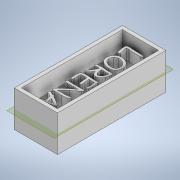
# Autodesk Inventor part: Pieza2
Saved by Autodesk Inventor 2021 (Build 250183000, 183)
## iProperties
Created: 2022-09-17
Part Number: Pieza2
Material: Genérico
Document SubType Name: Modeling
Designer: sergi
Density: 1 g/cm^3
Appearance: Valor por defecto
Author: sergi
Autodesk Inventor part; units mm, degrees
ref_plane "YZ Plane" through (0, 0, 0) normal (1, 0, 0) x (0, 1, 0)
ref_plane "XZ Plane" through (0, 0, 0) normal (0, 1, 0) x (-1, 0, 0)
ref_plane "XY Plane" through (0, 0, 0) normal (0, 0, 1) x (1, 0, 0)
sketch "Boceto1" plane through (0, 0, 0) normal (0, 1, 0) x (-1, 0, 0)
  line L0 (-6, -15) -> (6, -15)
  line L1 (6, -15) -> (6, 15)
  line L2 (6, 15) -> (-6, 15)
  line L3 (-6, 15) -> (-6, -15)
  line L4 (-6, -15) -> (6, 15) construction
  line L5 (6, -15) -> (-6, 15) construction
  line L6 (6, 15) -> (6, -15) construction
  line L7 (6, -15) -> (-6, -15) construction
  line L8 (-6, -15) -> (-6, 15) construction
  line L9 (-6, 15) -> (6, 15) construction
  point P0 (0, 0)
  dimension "d0" = 12
  dimension "d1" = 30
  dimension "d9" = 30
  dimension "d10" = 12
  constraints: 12 end point, 2 midpoint, 2 parallel, 1 horizontal, 1 perpendicular, 2 other
  measures "d0" distance of L2.end L1.end
  measures "d1" distance of L1.end L0.end
  measures "d9" distance of L7.end L9.start
  measures "d10" distance of L6.end L7.end
extrude "Extrusión1" add sketch "Boceto1" along normal blind 10
shell "Vaciado1" thickness 1 removed faces 1 at (2, 10, -5) ; own thickness 5 on faces at (2, 0, -5) ; own thickness 1 on faces at (2, 3.3333, -15)
sketch "Boceto2" plane through (-5, 5, 14) normal (0, 1, 0) x (1, 0, 0)
  line L0 (10.9835, 29) -> (10.9835, -1) construction
  line L1 (10.9835, -1) -> (-1.0165, -1) construction
  line L2 (-1.0165, -1) -> (-1.0165, 29) construction
  line L3 (-1.0165, 29) -> (10.9835, 29) construction
  line L4 (0, -2.0428) -> (0, 28)
  line L5 (-1, -1) -> (11, -1) projected
  spline S0 degree 2 poles (2.781, 23.9073) (2.6172, 24.2565) (2.4879, 25.0065) knots 0 0 0 1 1 1
  spline S1 degree 2 poles (2.4879, 25.0065) (2.3672, 25.6961) (2.3672, 26.1315) knots 0 0 0 1 1 1
  spline S2 degree 2 poles (2.3672, 26.1315) (2.3672, 26.4418) (2.462, 26.5797) knots 0 0 0 1 1 1
  spline S3 degree 2 poles (2.462, 26.5797) (2.5913, 26.7651) (2.9404, 26.7651) knots 0 0 0 1 1 1
  line L6 (2.9404, 26.7651) -> (3.962, 26.7047)
  spline S4 degree 2 poles (3.962, 26.7047) (5.3801, 26.6228) (7.1042, 26.6228) knots 0 0 0 1 1 1
  spline S5 degree 2 poles (7.1042, 26.6228) (7.2379, 26.6228) (7.4232, 26.4461) (7.4232, 26.3168) knots 0 0 0 1 2 2 2
  spline S6 degree 2 poles (7.4232, 26.3168) (7.4232, 26.1832) (7.2379, 26.0065) (7.1042, 26.0065) knots 0 0 0 1 2 2 2
  spline S7 degree 2 poles (7.1042, 26.0065) (5.3585, 26.0065) (3.9275, 26.0884) knots 0 0 0 1 1 1
  line L7 (3.9275, 26.0884) -> (3.4534, 26.1315)
  spline S8 degree 2 poles (3.4534, 26.1315) (3.1991, 26.153) (3.0008, 26.1487) knots 0 0 0 1 1 1
  spline S9 degree 2 poles (3.0008, 26.1487) (2.9922, 25.3427) (3.3758, 24.1099) knots 0 0 0 1 1 1
  spline S10 degree 2 poles (3.3758, 24.1099) (3.393, 24.0539) (3.393, 24.0108) knots 0 0 0 1 1 1
  spline S11 degree 2 poles (3.393, 24.0108) (3.393, 23.8772) (3.2896, 23.7866) knots 0 0 0 1 1 1
  spline S12 degree 2 poles (3.2896, 23.7866) (3.1948, 23.7091) (3.0698, 23.7091) knots 0 0 0 1 1 1
  spline S13 degree 2 poles (3.0698, 23.7091) (2.8715, 23.7091) (2.781, 23.9073) knots 0 0 0 1 1 1
  spline S14 degree 2 poles (2.4663, 21.1099) (2.4663, 21.9806) (2.9879, 22.5884) knots 0 0 0 1 1 1
  spline S15 degree 2 poles (2.9879, 22.5884) (3.5439, 23.2306) (4.4232, 23.2306) knots 0 0 0 1 1 1
  spline S16 degree 2 poles (4.4232, 23.2306) (5.4965, 23.2306) (6.3715, 22.597) knots 0 0 0 1 1 1
  spline S17 degree 2 poles (6.3715, 22.597) (7.3413, 21.8901) (7.3413, 20.8297) knots 0 0 0 1 1 1
  spline S18 degree 2 poles (7.3413, 20.8297) (7.3413, 19.8168) (6.8844, 19.3211) knots 0 0 0 1 1 1
  spline S19 degree 2 poles (6.8844, 19.3211) (6.406, 18.8039) (5.3801, 18.8039) knots 0 0 0 1 1 1
  spline S20 degree 2 poles (5.3801, 18.8039) (4.3111, 18.8039) (3.4491, 19.3858) knots 0 0 0 1 1 1
  spline S21 degree 2 poles (3.4491, 19.3858) (2.4663, 20.0539) (2.4663, 21.1099) knots 0 0 0 1 1 1
  spline S22 degree 2 poles (6.7077, 20.8297) (6.7077, 21.5884) (5.9534, 22.1142) knots 0 0 0 1 1 1
  spline S23 degree 2 poles (5.9534, 22.1142) (5.2594, 22.6013) (4.4232, 22.6013) knots 0 0 0 1 1 1
  spline S24 degree 2 poles (4.4232, 22.6013) (3.8284, 22.6013) (3.4534, 22.1573) knots 0 0 0 1 1 1
  spline S25 degree 2 poles (3.4534, 22.1573) (3.0999, 21.7349) (3.0999, 21.1099) knots 0 0 0 1 1 1
  spline S26 degree 2 poles (3.0999, 21.1099) (3.0999, 20.3599) (3.8585, 19.8685) knots 0 0 0 1 1 1
  spline S27 degree 2 poles (3.8585, 19.8685) (4.5353, 19.4332) (5.3801, 19.4332) knots 0 0 0 1 1 1
  spline S28 degree 2 poles (5.3801, 19.4332) (6.1215, 19.4332) (6.4189, 19.7651) knots 0 0 0 1 1 1
  spline S29 degree 2 poles (6.4189, 19.7651) (6.7077, 20.0797) (6.7077, 20.8297) knots 0 0 0 1 1 1
  spline S30 degree 2 poles (2.6215, 15.0496) (2.6215, 15.1659) (2.7206, 15.2694) knots 0 0 0 1 1 1
  spline S31 degree 2 poles (2.7206, 15.2694) (3.7292, 16.2909) (4.0784, 17.5453) knots 0 0 0 1 1 1
  line L8 (4.0784, 17.5453) -> (3.4749, 17.5194)
  line L9 (3.4749, 17.5194) -> (2.8672, 17.5022)
  spline S32 degree 2 poles (2.8672, 17.5022) (2.7292, 17.5022) (2.5482, 17.6789) (2.5482, 17.8125) knots 0 0 0 1 2 2 2
  spline S33 degree 2 poles (2.5482, 17.8125) (2.5482, 17.9461) (2.7292, 18.1228) (2.8672, 18.1228) knots 0 0 0 1 2 2 2
  spline S34 degree 2 poles (2.8672, 18.1228) (3.1129, 18.1228) (4.0784, 18.1703) (4.3241, 18.1703) knots 0 0 0 1 2 2 2
  spline S35 degree 2 poles (4.3241, 18.1703) (4.6085, 18.1703) (5.7335, 18.0453) (6.0137, 18.0453) knots 0 0 0 1 2 2 2
  spline S36 degree 2 poles (6.0137, 18.0453) (6.1732, 18.0453) (6.7896, 18.1056) (6.9491, 18.1056) knots 0 0 0 1 2 2 2
  spline S37 degree 2 poles (6.9491, 18.1056) (7.1258, 18.1056) (7.2594, 18.0065) knots 0 0 0 1 1 1
  spline S38 degree 2 poles (7.2594, 18.0065) (7.4232, 17.8901) (7.406, 17.6832) knots 0 0 0 1 1 1
  line L10 (7.406, 17.6832) -> (7.3456, 16.9375)
  spline S39 degree 2 poles (7.3456, 16.9375) (7.2939, 16.5151) (7.1387, 16.222) knots 0 0 0 1 1 1
  spline S40 degree 2 poles (7.1387, 16.222) (6.4749, 14.972) (5.518, 14.972) knots 0 0 0 1 1 1
  spline S41 degree 2 poles (5.518, 14.972) (5.0482, 14.972) (4.6861, 15.3987) knots 0 0 0 1 1 1
  spline S42 degree 2 poles (4.6861, 15.3987) (4.393, 15.7392) (4.2422, 16.2522) knots 0 0 0 1 1 1
  spline S43 degree 2 poles (4.2422, 16.2522) (3.7249, 15.2909) (3.1516, 14.8168) knots 0 0 0 1 1 1
  spline S44 degree 2 poles (3.1516, 14.8168) (3.0525, 14.7349) (2.9448, 14.7349) knots 0 0 0 1 1 1
  spline S45 degree 2 poles (2.9448, 14.7349) (2.8111, 14.7349) (2.6215, 14.9246) (2.6215, 15.0496) knots 0 0 0 1 2 2 2
  line L11 (6.7077, 17.0194) -> (6.7465, 17.4763)
  line L12 (6.7465, 17.4763) -> (6.3715, 17.4461)
  spline S46 degree 2 poles (6.3715, 17.4461) (6.143, 17.4246) (5.9965, 17.4246) knots 0 0 0 1 1 1
  spline S47 degree 2 poles (5.9965, 17.4246) (5.7508, 17.4246) (5.3801, 17.4634) knots 0 0 0 1 1 1
  line L13 (5.3801, 17.4634) -> (4.7637, 17.528)
  spline S48 degree 2 poles (4.7637, 17.528) (4.7637, 17.4849) (4.7594, 17.3039) (4.7594, 17.2565) knots 0 0 0 1 2 2 2
  spline S49 degree 2 poles (4.7594, 17.2565) (4.7594, 16.4677) (4.9706, 16.0754) knots 0 0 0 1 1 1
  spline S50 degree 2 poles (4.9706, 16.0754) (5.0654, 15.903) (5.2206, 15.7565) knots 0 0 0 1 1 1
  spline S51 degree 2 poles (5.2206, 15.7565) (5.393, 15.5927) (5.5137, 15.5927) knots 0 0 0 1 1 1
  spline S52 degree 2 poles (5.5137, 15.5927) (5.9448, 15.5927) (6.3154, 16.0797) knots 0 0 0 1 1 1
  spline S53 degree 2 poles (6.3154, 16.0797) (6.656, 16.528) (6.7077, 17.0194) knots 0 0 0 1 1 1
  spline S54 degree 2 poles (6.8154, 11.1056) (6.8154, 11.1487) (6.8327, 11.2047) knots 0 0 0 1 1 1
  spline S55 degree 2 poles (6.8327, 11.2047) (6.9792, 11.7263) (6.9792, 12.2134) knots 0 0 0 1 1 1
  spline S56 degree 2 poles (6.9792, 12.2134) (6.9792, 12.4634) (6.8887, 13.0668) (6.7939, 13.4116) knots 0 0 0 1 2 2 2
  spline S57 degree 2 poles (6.7939, 13.4116) (6.5913, 13.3815) (6.4706, 13.3815) knots 0 0 0 1 1 1
  spline S58 degree 2 poles (6.4706, 13.3815) (6.0439, 13.3815) (5.2896, 13.4375) knots 0 0 0 1 1 1
  line L14 (5.2896, 13.4375) -> (5.4189, 12.0797)
  spline S59 degree 2 poles (5.4189, 12.0797) (5.4792, 11.4849) (5.4792, 11.3513) knots 0 0 0 1 1 1
  spline S60 degree 2 poles (5.4792, 11.3513) (5.4792, 11.2134) (5.3068, 11.028) (5.1603, 11.028) knots 0 0 0 1 2 2 2
  spline S61 degree 2 poles (5.1603, 11.028) (4.8801, 11.028) (4.8456, 11.3125) knots 0 0 0 1 1 1
  line L15 (4.8456, 11.3125) -> (4.781, 12.0496)
  line L16 (4.781, 12.0496) -> (4.6516, 13.4806)
  spline S62 degree 2 poles (4.6516, 13.4806) (4.4318, 13.4935) (4.0396, 13.5065) (3.8715, 13.5065) knots 0 0 0 1 2 2 2
  spline S63 degree 2 poles (3.8715, 13.5065) (3.1861, 13.5065) (3.0654, 13.4073) knots 0 0 0 1 1 1
  spline S64 degree 2 poles (3.0654, 13.4073) (2.9792, 13.3341) (2.9792, 12.9203) knots 0 0 0 1 1 1
  spline S65 degree 2 poles (2.9792, 12.9203) (2.9792, 12.7306) (3.0008, 11.9591) (3.0008, 11.7651) knots 0 0 0 1 2 2 2
  spline S66 degree 2 poles (3.0008, 11.7651) (3.0008, 11.7047) (3.0396, 11.4634) (3.0396, 11.403) knots 0 0 0 1 2 2 2
  spline S67 degree 2 poles (3.0396, 11.403) (3.0396, 11.0754) (2.7206, 11.0754) knots 0 0 0 1 1 1
  spline S68 degree 2 poles (2.7206, 11.0754) (2.462, 11.0754) (2.4103, 11.3384) knots 0 0 0 1 1 1
  spline S69 degree 2 poles (2.4103, 11.3384) (2.3499, 11.6272) (2.3499, 12.597) knots 0 0 0 1 1 1
  spline S70 degree 2 poles (2.3499, 12.597) (2.3499, 13.5539) (2.6042, 13.8254) knots 0 0 0 1 1 1
  spline S71 degree 2 poles (2.6042, 13.8254) (2.8801, 14.1228) (3.8715, 14.1228) knots 0 0 0 1 1 1
  spline S72 degree 2 poles (3.8715, 14.1228) (4.0698, 14.1228) (4.5396, 14.1056) (4.8111, 14.0884) knots 0 0 0 1 2 2 2
  spline S73 degree 2 poles (4.8111, 14.0884) (4.8801, 14.1228) (4.962, 14.1228) knots 0 0 0 1 1 1
  spline S74 degree 2 poles (4.962, 14.1228) (5.0654, 14.1228) (5.1516, 14.0625) knots 0 0 0 1 1 1
  spline S75 degree 2 poles (5.1516, 14.0625) (6.0439, 14.0022) (6.4706, 14.0022) knots 0 0 0 1 1 1
  spline S76 degree 2 poles (6.4706, 14.0022) (6.587, 14.0022) (7.0266, 14.0625) (7.143, 14.0625) knots 0 0 0 1 2 2 2
  spline S77 degree 2 poles (7.143, 14.0625) (7.5094, 14.0625) (7.5094, 13.7522) knots 0 0 0 1 1 1
  spline S78 degree 2 poles (7.5094, 13.7522) (7.5094, 13.6228) (7.4189, 13.5323) knots 0 0 0 1 1 1
  spline S79 degree 2 poles (7.4189, 13.5323) (7.518, 13.1616) (7.6172, 12.5022) (7.6172, 12.2091) knots 0 0 0 1 2 2 2
  spline S80 degree 2 poles (7.6172, 12.2091) (7.6172, 11.4591) (7.4361, 11.0108) knots 0 0 0 1 1 1
  spline S81 degree 2 poles (7.4361, 11.0108) (7.3542, 10.8039) (7.1387, 10.8039) knots 0 0 0 1 1 1
  spline S82 degree 2 poles (7.1387, 10.8039) (7.018, 10.8039) (6.9189, 10.8858) knots 0 0 0 1 1 1
  spline S83 degree 2 poles (6.9189, 10.8858) (6.8154, 10.972) (6.8154, 11.1056) knots 0 0 0 1 1 1
  spline S84 degree 2 poles (3.3413, 5.8341) (3.1948, 5.8341) (2.8456, 5.8858) knots 0 0 0 1 1 1
  spline S85 degree 2 poles (2.8456, 5.8858) (2.5353, 5.9332) (2.5353, 6.2134) knots 0 0 0 1 1 1
  spline S86 degree 2 poles (2.5353, 6.2134) (2.5353, 6.3858) (2.7594, 6.6228) knots 0 0 0 1 1 1
  spline S87 degree 2 poles (2.7594, 6.6228) (3.9491, 7.8772) (6.1948, 9.5065) knots 0 0 0 1 1 1
  line L17 (6.1948, 9.5065) -> (5.4922, 9.5237)
  line L18 (5.4922, 9.5237) -> (4.7853, 9.5323)
  spline S88 degree 2 poles (4.7853, 9.5323) (4.531, 9.5323) (3.5008, 9.5108) (3.2422, 9.5108) knots 0 0 0 1 2 2 2
  spline S89 degree 2 poles (3.2422, 9.5108) (2.4103, 9.5108) (2.4103, 9.8341) knots 0 0 0 1 1 1
  spline S90 degree 2 poles (2.4103, 9.8341) (2.4103, 10.0022) (2.518, 10.1013) knots 0 0 0 1 1 1
  spline S91 degree 2 poles (2.518, 10.1013) (2.6129, 10.1918) (2.7465, 10.1918) knots 0 0 0 1 1 1
  spline S92 degree 2 poles (2.7465, 10.1918) (2.8758, 10.1918) (3.4016, 10.153) (3.5353, 10.153) knots 0 0 0 1 2 2 2
  spline S93 degree 2 poles (3.5353, 10.153) (3.7249, 10.153) (4.4879, 10.1272) (4.6818, 10.1272) knots 0 0 0 1 2 2 2
  spline S94 degree 2 poles (4.6818, 10.1272) (4.8844, 10.1272) (5.712, 10.1444) (5.9146, 10.1444) knots 0 0 0 1 2 2 2
  spline S95 degree 2 poles (5.9146, 10.1444) (6.1085, 10.1444) (6.8801, 10.222) (7.0741, 10.222) knots 0 0 0 1 2 2 2
  spline S96 degree 2 poles (7.0741, 10.222) (7.2163, 10.222) (7.4534, 9.9763) (7.4534, 9.8211) knots 0 0 0 1 2 2 2
  spline S97 degree 2 poles (7.4534, 9.8211) (7.4534, 9.6573) (7.0956, 9.4159) knots 0 0 0 1 1 1
  spline S98 degree 2 poles (7.0956, 9.4159) (5.9404, 8.6444) (5.1775, 8.0323) knots 0 0 0 1 1 1
  spline S99 degree 2 poles (5.1775, 8.0323) (4.2723, 7.2996) (3.4448, 6.4246) knots 0 0 0 1 1 1
  spline S100 degree 2 poles (3.4448, 6.4246) (3.5784, 6.4159) (3.837, 6.4246) knots 0 0 0 1 1 1
  line L19 (3.837, 6.4246) -> (4.2249, 6.4332)
  spline S101 degree 2 poles (4.2249, 6.4332) (5.5827, 6.4332) (6.3887, 6.5366) knots 0 0 0 1 1 1
  spline S102 degree 2 poles (6.3887, 6.5366) (6.4663, 6.5496) (6.712, 6.6228) knots 0 0 0 1 1 1
  spline S103 degree 2 poles (6.712, 6.6228) (6.9232, 6.6832) (7.0396, 6.6832) knots 0 0 0 1 1 1
  spline S104 degree 2 poles (7.0396, 6.6832) (7.3973, 6.6832) (7.3973, 6.3556) knots 0 0 0 1 1 1
  spline S105 degree 2 poles (7.3973, 6.3556) (7.3973, 5.8168) (5.393, 5.8168) knots 0 0 0 1 1 1
  spline S106 degree 2 poles (5.393, 5.8168) (5.0482, 5.8168) (3.6861, 5.8341) (3.3413, 5.8341) knots 0 0 0 1 2 2 2
  spline S107 degree 2 poles (2.5611, 1.6875) (2.5611, 1.972) (3.2896, 2.1832) knots 0 0 0 1 1 1
  spline S108 degree 2 poles (3.2896, 2.1832) (3.5698, 2.2651) (4.2637, 2.3858) knots 0 0 0 1 1 1
  spline S109 degree 2 poles (4.2637, 2.3858) (4.2206, 2.7004) (4.1085, 3.2091) knots 0 0 0 1 1 1
  line L20 (4.1085, 3.2091) -> (3.9404, 4.028)
  spline S110 degree 2 poles (3.9404, 4.028) (3.5353, 4.1832) (2.7551, 4.5625) knots 0 0 0 1 1 1
  spline S111 degree 2 poles (2.7551, 4.5625) (2.5827, 4.6616) (2.5827, 4.8297) knots 0 0 0 1 1 1
  spline S112 degree 2 poles (2.5827, 4.8297) (2.5827, 4.9547) (2.7637, 5.1487) (2.893, 5.1487) knots 0 0 0 1 2 2 2
  spline S113 degree 2 poles (2.893, 5.1487) (3.0439, 5.1487) (4.0223, 4.6832) knots 0 0 0 1 1 1
  spline S114 degree 2 poles (4.0223, 4.6832) (4.1042, 4.7349) (4.2077, 4.7349) knots 0 0 0 1 1 1
  spline S115 degree 2 poles (4.2077, 4.7349) (4.4577, 4.7349) (4.531, 4.4332) knots 0 0 0 1 1 1
  spline S116 degree 2 poles (4.531, 4.4332) (5.1904, 4.0797) (6.0525, 3.5409) knots 0 0 0 1 1 1
  spline S117 degree 2 poles (6.0525, 3.5409) (7.2249, 2.8082) (7.2249, 2.6272) knots 0 0 0 1 1 1
  spline S118 degree 2 poles (7.2249, 2.6272) (7.2249, 2.3858) (6.8844, 2.2953) knots 0 0 0 1 1 1
  line L21 (6.8844, 2.2953) -> (5.8456, 2.1013)
  line L22 (5.8456, 2.1013) -> (3.6948, 1.6401)
  line L23 (3.6948, 1.6401) -> (3.2077, 1.4634)
  spline S119 degree 2 poles (3.2077, 1.4634) (2.9577, 1.3728) (2.8715, 1.3728) knots 0 0 0 1 1 1
  spline S120 degree 2 poles (2.8715, 1.3728) (2.7422, 1.3728) (2.5611, 1.5625) (2.5611, 1.6875) knots 0 0 0 1 2 2 2
  line L24 (6.0956, 2.778) -> (4.6689, 3.6616)
  spline S121 degree 2 poles (4.6689, 3.6616) (4.7637, 3.2866) (4.9016, 2.528) knots 0 0 0 1 1 1
  line L25 (4.9016, 2.528) -> (6.0956, 2.778)
  point P0 (5, 14)
  dimension "d7" = 30
  dimension "d8" = 12
  constraints: 2 end point, 1 collinear, 2 other
  measures "d7" distance of L1.end L2.end
  measures "d8" distance of L0.end L1.end
ref_plane "Plano de trabajo2" through (0, 5, 0) normal (0, -1, 0) x (1, 0, 0)
extrude "Extrusión2" add sketch "Boceto2" along normal blind 3
